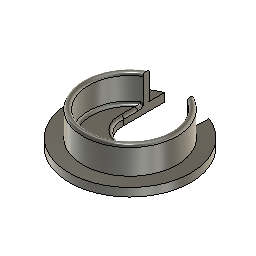
base_cable_cover v2 (Autodesk Fusion 360 design; units mm, degrees)
Autodesk Fusion 360 part; units mm, degrees
note: some values were not read from the file. Set by a fixed rule: which sketch regions a step uses.
sketch "Sketch1" plane through (0, 0, 0) normal (0, 0, 1) x (1, 0, 0) in component "base_cable_cover"
  circle A0 centre (0, 0) radius 11
  dimension "d1" = 22
  constraint coincident A0.centre origin
  measures "d1" diameter of A0
extrude "Extrude1" add sketch "Sketch1" along normal blind 1.5 in component "base_cable_cover"
sketch "Sketch2" plane through (0, 0, 1.5) normal (0, 0, 1) x (-1, 0, 0) in component "base_cable_cover"
  circle A0 centre (0, 0) radius 11
  circle A1 centre (0, 0) radius 8.5
  circle A2 centre (0, 0) radius 7.5
  dimension "d4" = 17
  dimension "d7" = 15
  constraint coincident A0.centre A1.centre
  constraint concentric A1 A2
  measures "d4" diameter of A1
  measures "d7" diameter of A2
extrude "Extrude2" add sketch "Sketch2" along normal blind 5 contours A1 in component "base_cable_cover"
sketch "Sketch3" plane through (0, 0, 1.5) normal (0, 0, 1) x (-1, 0, 0) in component "base_cable_cover"
  circle A0 centre (0, 0) radius 7.5
  line L0 (0, 0) -> (11, 0) construction
  circle A1 centre (0, 0) radius 8.5
  line L1 (4, -6.3443) -> (4, -2.8443)
  line L2 (0, 0) -> (0, -11.235) construction
  line L3 (0, -11.235) -> (0, -5) construction
  line L4 (-4, -6.3443) -> (-4, -2.8443)
  arc A2 (4, -2.8443) -> (-4, -2.8443) centre (0, -2.5441) ccw
  point P0 (11, 0)
  dimension "d12" = 4
  dimension "d13" = 3.5
  constraint coincident A0.centre L0.start
  constraint coincident P0 L0.end
  constraint coincident A0 L1.start
  constraint vertical L1
  constraint vertical L2
  constraint coincident L2 L3.end
  constraint symmetric L1.start L2 L4.start
  constraint symmetric L1.end L2 L4.end
  measures "d12" distance of L1 L2
  measures "d13" distance of L1.start L1.end
extrude "Extrude3" cut sketch "Sketch3" against normal blind 16 contours A0 L1 L4 A2 picked at (0, -4.3962) in component "base_cable_cover"
fillet "Fillet1" radius 0.5 6 edges at (7.9248, 3.0737, 6.5) (6.9925, -2.7121, 6.5) (0, -7.5, 1.5) (0, -1.4671, 1.5) (-4, 4.5943, 1.5) (4, 4.5943, 1.5) in component "base_cable_cover"
sketch "Sketch4" plane through (0, 0, 0) normal (0, 0, -1) x (1, 0, 0) in component "base_cable_cover"
  line L0 (-4, -6.3443) -> (-4, -2.8443)
  arc A0 (4, -2.8443) -> (-4, -2.8443) centre (0, -2.5441) ccw
  line L1 (4, -2.8443) -> (4, -6.3443)
  arc A1 (-4, -6.3443) -> (4, -6.3443) centre (0, 0) ccw
  circle A2 centre (0, 0) radius 11
  line L2 (-4, -6.3443) -> (-4, -13)
  line L3 (4, -6.3443) -> (4.2188, -12.7648)
  line L4 (4.2188, -12.7648) -> (-4, -12.7648)
  constraint coincident L0.start A1.start
  constraint parallel L0 L2
  constraint coincident L1.end A1.end
  constraint coincident L2 L4.end
  constraint perpendicular L2 L4
extrude "Extrude4" cut sketch "Sketch4" against normal blind 8 contours A1 A2 L2 L3 | A2 L2 L3 L4 in component "base_cable_cover"
component "base_cable_cover" placed x (1, 0, 0) y (0, 1, 0) z (0, 0, 1) at (0, 0, 0)
